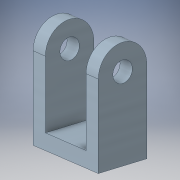
# Autodesk Inventor part: Base_Block
Saved by Autodesk Inventor 2016 (Build 200138000, 138)
## iProperties
Created: 2017-07-15
Part Number: Base_Block
Material: Steel, Carbon
Document SubType Name: Modeling
Designer: bobbyl
Density: 7.85 g/cm^3
Appearance: Steel Blue
Author: bobbyl
Autodesk Inventor part; units mm, degrees
ref_plane "YZ Plane" through (0, 0, 0) normal (1, 0, 0) x (0, 1, 0)
ref_plane "XZ Plane" through (0, 0, 0) normal (0, 1, 0) x (-1, 0, 0)
ref_plane "XY Plane" through (0, 0, 0) normal (0, 0, 1) x (1, 0, 0)
sketch "Sketch1" plane through (0, 0, 0) normal (0, 1, 0) x (-1, 0, 0)
  line L0 (56, 0) -> (-56, 0) projected
  line L1 (0, -35) -> (0, 35) projected
  line L2 (40, 25) -> (-40, 25)
  line L3 (-40, 25) -> (-40, -25)
  line L4 (-40, -25) -> (40, -25)
  line L5 (40, -25) -> (40, 25)
  point P0 (0, 0)
  point P1 (40, 0)
  point P2 (0, -25)
  dimension "d0" = 50
  dimension "d1" = 80
  constraints: 8 end point, 2 midpoint, 2 parallel, 2 point on line, 1 horizontal, 1 perpendicular
  measures "d0" distance of L4.end L2.start
  measures "d1" distance of L3.end L4.end
extrude "Extrusion1" add sketch "Sketch1" along normal blind 15
sketch "Sketch2" plane through (40, 0, 25) normal (1, 0, 0) x (0, 0, -1)
  line L0 (0, 0) -> (50, 0) projected
  line L1 (50, 0) -> (50, 15) projected
  line L2 (0, 15) -> (50, 15) projected
  line L3 (0, 0) -> (0, 15) projected
  line L4 (0, 0) -> (50, 0)
  line L5 (50, 0) -> (50, 80)
  line L6 (0, 80) -> (0, 0)
  arc A0 (50, 80) -> (0, 80) centre (25, 80) ccw
  line L7 (0, 0) -> (50, 0) projected
  circle A1 centre (25, 80) radius 10
  line L8 (25, -19) -> (25, 114) projected
  point P0 (25, 0)
  dimension "d5" = 50
  dimension "d6" = 20
  dimension "d7" = 80
  dimension "d8" = 50
  constraints: 6 end point, 2 centre point, 2 point on circle, 2 point on line, 1 coincident, 1 collinear, 1 horizontal, 1 parallel, 1 perpendicular
  measures "d5" diameter of A0
  measures "d6" diameter of A1
  measures "d7" distance of L6.start L4.start
  measures "d8" distance between parallel lines of L5 L6
extrude "Extrusion2" add sketch "Sketch2" against normal blind 15 contours L3 L2 L8 L0 | L8 L2 L1 L0 | L6 A0 L8 A1 L2 | L8 A1 A0 L5 L2
mirror "Mirror1" about plane through (0, 0, 0) normal (1, 0, 0) of "Extrusion2"
body "Solid1"
